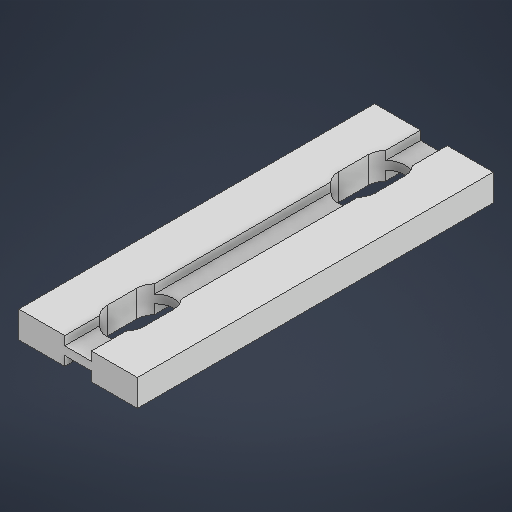
# Autodesk Inventor part: Spacer Laser
Saved by Autodesk Inventor 2025 (Build 290162000, 162)
## iProperties
Created: 2024-07-08
Part Number: Spacer Laser
Material: Generic
Document SubType Name: Modeling
Designer: mayhe
Density: 1 g/cm^3
Appearance: Default
Author: mayhe
Autodesk Inventor part; units mm, degrees
ref_plane "YZ Plane" through (0, 0, 0) normal (1, 0, 0) x (0, 1, 0)
ref_plane "XZ Plane" through (0, 0, 0) normal (0, 1, 0) x (-1, 0, 0)
ref_plane "XY Plane" through (0, 0, 0) normal (0, 0, 1) x (1, 0, 0)
sketch "Sketch1" plane through (0, 0, 0) normal (0, 0, 1) x (1, 0, 0)
  line L0 (-10, 2.25) -> (10, 2.25)
  line L1 (10, 2.25) -> (10, -2.25)
  line L2 (10, -2.25) -> (-10, -2.25)
  line L3 (-10, -2.25) -> (-10, 2.25)
  line L4 (-10, 2.25) -> (10, -2.25) construction
  line L5 (10, 2.25) -> (-10, -2.25) construction
  line L6 (-2.25, 3.75) -> (2.25, 3.75)
  line L7 (2.25, 3.75) -> (2.25, 0.75)
  line L8 (2.25, 0.75) -> (-2.25, 0.75)
  line L9 (-2.25, 0.75) -> (-2.25, 3.75)
  line L10 (-2.25, 3.75) -> (2.25, 0.75) construction
  line L11 (2.25, 3.75) -> (-2.25, 0.75) construction
  line L12 (-2.25, -0.6661) -> (2.25, -0.6661)
  line L13 (2.25, -0.6661) -> (2.25, -3.8339)
  line L14 (2.25, -3.8339) -> (-2.25, -3.8339)
  line L15 (-2.25, -3.8339) -> (-2.25, -0.6661)
  line L16 (-2.25, -0.6661) -> (2.25, -3.8339) construction
  line L17 (2.25, -0.6661) -> (-2.25, -3.8339) construction
  point P0 (0, 0)
  point P1 (0, 2.25)
  point P2 (0, -2.25)
  point P3 (2.25, 2.25)
  point P4 (-2.25, 2.25)
  point P5 (-2.25, -2.25)
  point P6 (2.25, -2.25)
  dimension "d0" = 20
  dimension "d1" = 4.5
  dimension "d2" = 4.5
  dimension "d3" = 3
  constraints: 36 end point, 8 midpoint, 6 parallel, 3 horizontal, 3 perpendicular, 1 point on line
  measures "d0" distance of L1.end L2.end
  measures "d1" distance of L0.end L1.end
  measures "d2" distance of L7.end L8.end
  measures "d3" distance of L6.end L7.end
extrude "Extrusion1" add sketch "Sketch1" along normal mid plane 60 contours L0 L9 L8 L7 L1 L2 L13 L12 L15 L3
sketch "Sketch2" plane through (2.25, 2.25, 30) normal (0, 1, 0) x (1, 0, 0)
  line L0 (-5.35, 13) -> (0.85, 13)
  line L1 (0.85, 13) -> (0.85, 8)
  line L2 (0.85, 8) -> (-5.35, 8)
  line L3 (-5.35, 8) -> (-5.35, 13)
  line L4 (-5.35, 13) -> (0.85, 8) construction
  line L5 (0.85, 13) -> (-5.35, 8) construction
  line L6 (0, 0) -> (-4.5, 0) projected
  circle A0 centre (-2.25, 8) radius 3.1
  circle A1 centre (-2.25, 13) radius 3.1
  line L7 (7.75, 0) -> (7.75, 60) projected
  line L8 (7.75, 30) -> (-12.25, 30)
  line L9 (-12.25, 60) -> (-12.25, 0) projected
  line L10 (0.85, 47) -> (0.85, 52)
  line L11 (-5.35, 52) -> (-5.35, 47)
  circle A2 centre (-2.25, 52) radius 3.1
  circle A3 centre (-2.25, 47) radius 3.1
  point P0 (-2.25, 30)
  point P1 (-2.25, 10.5)
  point P2 (-2.25, 49.5)
  dimension "d6" = 6.2
  dimension "d7" = 5
  dimension "d8" = 8
  constraints: 18 end point, 8 symmetric about line, 6 midpoint, 3 horizontal, 2 coincident, 2 parallel, 1 perpendicular, 12 other
  measures "d6" distance of L1.end L2.end
  measures "d7" distance of L0.end L1.end
  measures "d8" distance from line of L6 point (-2.25, 8)
extrude "Extrusion2" cut sketch "Sketch2" against normal blind 60
body "Solid1"
